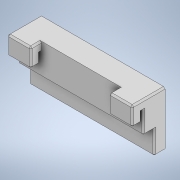
# Autodesk Inventor part: euro_box_center
Saved by Autodesk Inventor 2020 (Build 240168000, 168)
## iProperties
Created: 2019-11-19
Part Number: euro_box_center
Material: Generic
Document SubType Name: Modeling
Designer: NILY
Density: 1 g/cm^3
Appearance: Default
Author: NILY
Autodesk Inventor part; units mm, degrees
ref_plane "YZ Plane" through (0, 0, 0) normal (1, 0, 0) x (0, 1, 0)
ref_plane "XZ Plane" through (0, 0, 0) normal (0, 1, 0) x (-1, 0, 0)
ref_plane "XY Plane" through (0, 0, 0) normal (0, 0, 1) x (1, 0, 0)
sketch "Sketch1" plane through (0, 0, 0) normal (0, 0, 1) x (1, 0, 0)
  line L0 (0, 0) -> (80, 0)
  line L1 (80, 0) -> (80, -20)
  line L2 (80, -20) -> (0, -20)
  line L3 (0, -20) -> (0, 0)
  dimension "d0" = 80
  dimension "d1" = 20
  constraints: 8 end point, 2 parallel, 1 horizontal, 1 perpendicular
  measures "d0" distance of L1.end L2.end
  measures "d1" distance of L0.end L1.end
extrude "Extrusion1" add sketch "Sketch1" along normal blind 7
sketch "Sketch2" plane through (0, 0, 7) normal (0, 0, 1) x (1, 0, 0)
  line L0 (0, 0) -> (80, 0)
  line L1 (80, 0) -> (80, -5)
  line L2 (80, -5) -> (0, -5)
  line L3 (0, -5) -> (0, 0)
  dimension "d4" = 80
  dimension "d5" = 5
  constraints: 8 end point, 2 parallel, 1 horizontal, 1 perpendicular
  measures "d4" distance of L1.end L2.end
  measures "d5" distance of L0.end L1.end
extrude "Extrusion2" add sketch "Sketch2" along normal blind 7
sketch "Sketch3" plane through (0, -5, 7) normal (0, -1, 0) x (1, 0, 0)
  line L0 (0, -7) -> (0, 7) projected
  line L1 (0, 7) -> (80, 7)
  line L2 (80, 7) -> (80, 2)
  line L3 (80, 2) -> (0, 2)
  line L4 (0, 2) -> (0, 7)
  dimension "d8" = 80
  dimension "d9" = 5
  constraints: 8 end point, 2 parallel, 1 horizontal, 1 perpendicular
  measures "d8" distance of L2.end L3.end
  measures "d9" distance of L1.end L2.end
extrude "Extrusion3" add sketch "Sketch3" along normal blind 7
sketch "Sketch6" plane through (0, 0, 14) normal (0, 0, 1) x (1, 0, 0)
  line L0 (80, 0) -> (0, 0) projected
  line L1 (1, -12) -> (79, -12) projected
  line L2 (15, 0) -> (65, 0)
  line L3 (65, 0) -> (65, -12)
  line L4 (65, -12) -> (15, -12)
  line L5 (15, -12) -> (15, 0)
  line L6 (0, -1) -> (0, -11) projected
  point P0 (79, 0)
  point P1 (1, 0)
  dimension "d28" = 50
  dimension "d29" = 15
  constraints: 8 end point, 2 parallel, 2 point on line, 1 horizontal, 1 perpendicular
  measures "d28" distance of L3.end L4.end
  measures "d29" distance between parallel lines of L6 L5
extrude "Extrusion6" cut sketch "Sketch6" against normal blind 7
sketch "Sketch7" plane through (0, 0, 0) normal (0, 0, -1) x (-1, 0, 0)
  line L0 (0, 0) -> (-80, 0)
  line L1 (-80, 0) -> (-80, -35)
  line L2 (-80, -35) -> (0, -35)
  line L3 (0, -35) -> (0, 0)
  dimension "d38" = 80
  dimension "d39" = 35
  constraints: 8 end point, 2 parallel, 1 horizontal, 1 perpendicular
  measures "d38" distance of L2.end L1.end
  measures "d39" distance of L1.end L0.end
extrude "Extrusion7" add sketch "Sketch7" along normal blind 7
sketch "Sketch8" plane through (0, 0, -7) normal (0, 0, -1) x (-1, 0, 0)
  circle A0 centre (-20, -17.75) radius 2.5
  line L0 (0, 0) -> (-80, 0) projected
  line L1 (0, -35) -> (0, 0) projected
  dimension "d42" = 5
  dimension "d43" = 17.75
  dimension "d44" = 20
  constraints: 1 centre point
  measures "d42" diameter of A0
  measures "d43" distance from line of L0 A0.centre
  measures "d44" distance from line of L1 A0.centre
extrude "Extrusion8" add sketch "Sketch8" along normal blind 5
sketch "Sketch9" plane through (0, 0, -7) normal (0, 0, -1) x (-1, 0, 0)
  circle A0 centre (-60, -17.75) radius 2.5
  line L0 (0, 0) -> (-80, 0) projected
  line L1 (-80, 0) -> (-80, -35) projected
  dimension "d47" = 5
  dimension "d48" = 17.75
  dimension "d49" = 20
  constraints: 1 centre point
  measures "d47" diameter of A0
  measures "d48" distance from line of L0 A0.centre
  measures "d49" distance from line of L1 A0.centre
extrude "Extrusion9" add sketch "Sketch9" along normal blind 5
chamfer "Chamfer5" distance 1 angle 45 30 edges at (0, -35, -3.5) (0, -27.5, 0) (0, -20, 3.5) (0, -12.5, 7) (40, -20, 7) (40, -35, 0) (0, 0, 3.5) (22.5, -17.75, -12) (62.5, -17.75, -12) (0, -6, 14) (72.5, -12, 14) (7.5, -12, 14) (15, -6, 14) (7.5, 0, 14) (7.5, -12, 9) (0, -12, 11.5) (15, -12, 11.5) (65, 0, 10.5) (65, -6, 14) (65, -12, 11.5) (72.5, -12, 9) (80, -12, 11.5) (80, -6, 14) (72.5, 0, 14) (80, 0, 3.5) (80, -35, -3.5) (80, -27.5, 0) (80, -20, 3.5) (80, -12.5, 7) (15, 0, 10.5)
body "Solid1"
